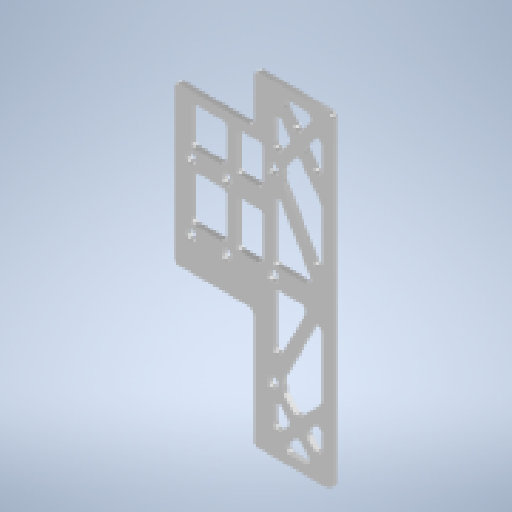
# Autodesk Inventor part: base2fork_connecter_front
Saved by Autodesk Inventor 2024.1 (Build 281209000, 209)
## iProperties
Created: 2025-03-04
Part Number: base2fork_connecter_front
Material: アルミニウム 6061
Document SubType Name: Sheet Metal
Designer: hibik
Density: 2.7 g/cm^3
Sheet Metal Rule: Default_mm
Appearance: アルミニウム - フラット
Author: hibik
Autodesk Inventor part; units mm, degrees
ref_plane "YZ Plane" through (0, 0, 0) normal (1, 0, 0) x (0, 1, 0)
ref_plane "XZ Plane" through (0, 0, 0) normal (0, 1, 0) x (-1, 0, 0)
ref_plane "XY Plane" through (0, 0, 0) normal (0, 0, 1) x (1, 0, 0)
sketch "スケッチ1 outline for プレート1" plane through (0, 0, 0) normal (0, 0, 1) x (1, 0, 0)
  line L0 (11.969655, 0) -> (24.990381, 0)
  line L1 (4.255354, 0) -> (11.969655, 0)
  line L2 (24.990381, 0) -> (24.990381, 47.7)
  line L3 (4.255354, 47.7) -> (4.255354, 0)
  line L4 (24.990381, 47.7) -> (13.490381, 47.7)
  line L5 (13.490381, 47.7) -> (4.255354, 47.7)
  circle A0 centre (9.255354, 10) radius 1.6
  circle A1 centre (19.990381, 10) radius 1.6
  circle A2 centre (9.255354, 30) radius 1.6
  circle A3 centre (19.990381, 30) radius 1.6
extrude "プレート1" add sketch "スケッチ1 outline for プレート1" along normal blind 1.5
sketch "スケッチ2 outline for プレート2" plane through (0, 0, 1.5) normal (0, 0, 1) x (1, 0, 0)
  line L0 (28.216878, 0) -> (28.216878, -35.8)
  line L1 (28.216878, -35.8) -> (51.990381, -35.8)
  line L2 (51.990381, -35.8) -> (51.990381, 62.7)
  line L3 (51.990381, 62.7) -> (28.216878, 62.7)
  line L4 (28.216878, 62.7) -> (28.216878, 47.7)
  line L5 (28.216878, 47.7) -> (24.990381, 47.7)
  line L6 (24.990381, 47.7) -> (24.990381, 0)
  line L7 (24.990381, 0) -> (28.216878, 0)
  circle A0 centre (33.990381, -16.45) radius 1.6
  circle A1 centre (33.990381, 39.55) radius 1.6
  circle A2 centre (33.990381, 11.55) radius 1.6
sheet face with bend "面2" sketch "スケッチ2 outline for プレート2" thickness 1.5 toward (0, 0, -1) bend radius 1.5
bend "曲げ1"
sketch "スケッチ1" plane through (0, 0, 0) normal (0, 0, 1) x (1, 0, 0)
  circle A0 centre (9.255354, 10) radius 1.6
  circle A1 centre (19.990381, 30) radius 1.6
  circle A2 centre (9.255354, 30) radius 1.6
  circle A3 centre (19.990381, 50) radius 1.6
  circle A4 centre (19.990381, 10) radius 1.6
  line L0 (13.490381, 47.7) -> (-5.744646, 47.7)
  line L1 (-5.744646, 47.7) -> (-5.744646, 0)
  line L2 (0, 0) -> (-5.744646, 0)
  line L3 (0, -16) -> (0, 0)
  line L4 (0, -16) -> (11.969655, -16)
  line L5 (11.969655, 0) -> (11.969655, -16)
  line L6 (24.990381, 0) -> (11.969655, 0)
  line L7 (24.990381, 62.7) -> (24.990381, 0)
  line L8 (13.490381, 62.7) -> (24.990381, 62.7)
  line L9 (13.490381, 62.7) -> (13.490381, 47.7)
  line L10 (0, 0) -> (11.969655, 0)
  line L11 (4.255354, 47.7) -> (4.255354, 0)
  line L12 (13.490381, 47.7) -> (24.990381, 47.7)
  dimension "d0" = 5
  dimension "d1" = 15
  dimension "d2" = 20
  dimension "d3" = 20
  dimension "d4" = 10
  dimension "d5" = 30.73503
  dimension "d6" = 78.7
  dimension "d7" = 62.7
  dimension "d8" = 19.23503
  dimension "d9" = 11.96966
  dimension "d10" = 5.74465
  dimension "d11" = 15
  dimension "d12" = 3.2
  dimension "d14" = 5
  measures "d0" distance from line of L7 A3.centre
  measures "d1" distance from line of L1 A2.centre
  measures "d2" distance of A1.centre A3.centre
  measures "d3" distance of A4.centre A1.centre
  measures "d4" distance from line of L6 A4.centre
  measures "d5" distance between parallel lines of L1 L7
  measures "d6" distance between parallel lines of L4 L8
  measures "d7" distance of L7.start L6.start
  measures "d8" distance of L0.start L0.end
  measures "d9" distance of L3.start L4.end
  measures "d10" distance of L2.start L1.end
  measures "d11" distance of L8.start L0.start
  measures "d12" diameter of A3
  measures "d14" distance from line of L11 A2.centre
sketch "スケッチ2" plane through (0, 0, 1.5) normal (0, 0, 1) x (1, 0, 0)
  circle A0 centre (33.990381, 39.55) radius 1.6
  circle A1 centre (33.990381, 11.55) radius 1.6
  circle A2 centre (33.990381, -16.45) radius 1.6
  line L0 (28.216878, -34.3) -> (51.990381, -34.3)
  line L1 (51.990381, -34.3) -> (51.990381, 62.7)
  line L2 (28.216878, 62.7) -> (51.990381, 62.7)
  line L3 (28.216878, -34.3) -> (28.216878, 62.7)
  line L4 (39.417474, -31.3) -> (32.835681, -31.3)
  line L5 (32.835681, -31.3) -> (32.835681, -27.3)
  line L6 (32.835681, -27.3) -> (39.417474, -27.3)
  line L7 (39.417474, -27.3) -> (39.417474, -31.3)
  line L8 (39.417474, 59.7) -> (39.417474, 55.7)
  line L9 (39.417474, 55.7) -> (32.835681, 55.7)
  line L10 (32.835681, 55.7) -> (32.835681, 59.7)
  line L11 (39.417474, 59.7) -> (32.835681, 59.7)
  line L12 (24.990381, 47.7) -> (24.990381, 0)
  line L13 (24.990381, 0) -> (28.216878, 0)
  line L14 (28.216878, -34.3) -> (51.990381, -34.3)
  line L15 (51.990381, -34.3) -> (51.990381, -35.8)
  line L16 (51.990381, -35.8) -> (28.216878, -35.8)
  line L17 (28.216878, -35.8) -> (28.216878, -34.3)
  line L18 (30.216878, 0) -> (30.216878, -35.8)
  line L19 (4.255354, 0) -> (24.990381, 0)
  line L20 (24.990381, 0) -> (30.216878, 0)
  line L21 (24.990381, 47.7) -> (28.216878, 47.7)
  point P0 (0, 0)
  point P1 (30.216878, -34.3)
  dimension "d21" = 1.5
  dimension "d25" = 2
  measures "d21" distance of L14.end L15.end
  measures "d25" distance between parallel lines of L3 L18
fillet "フィレット1" radius 1.5 4 edges at (4.2554, 0, 0.75) (4.2554, 47.7, 0.75) (51.9904, 62.7, 0.75) (51.9904, -35.8, 0.75)
sketch "スケッチ3" plane through (0, 0, 1.5) normal (0, 0, 1) x (1, 0, 0)
  arc A0 (5.755354, 47.7) -> (4.255354, 46.2) centre (5.755354, 46.2) ccw
  line L0 (4.255354, 1.5) -> (4.255354, 46.2)
  arc A1 (4.255354, 1.5) -> (5.755354, 0) centre (5.755354, 1.5) ccw
  line L1 (28.216878, 0) -> (5.755354, 0)
  circle A2 centre (19.990381, 10) radius 1.6
  circle A3 centre (9.255354, 30) radius 1.6
  circle A4 centre (19.990381, 30) radius 1.6
  circle A5 centre (9.255354, 10) radius 1.6
  line L2 (19.990381, 10) -> (9.255354, 10)
  line L3 (9.255354, 10) -> (9.255354, 44.7)
  line L4 (9.255354, 44.7) -> (19.990381, 44.7)
  line L5 (19.990381, 44.7) -> (19.990381, 10)
  circle A6 centre (9.255354, 30) radius 3
  circle A7 centre (19.990381, 30) radius 3
  circle A8 centre (19.990381, 10) radius 3
  circle A9 centre (9.255354, 10) radius 3
  line L6 (33.990381, 59.7) -> (48.990381, 59.7)
  line L7 (48.990381, 59.7) -> (48.990381, -32.8)
  line L8 (48.990381, -32.8) -> (33.990381, -32.8)
  line L9 (33.990381, -32.8) -> (33.990381, 59.7)
  line L10 (32.885071, -31.785954) -> (35.095691, -33.814046)
  line L11 (35.095691, -33.814046) -> (50.095691, -17.464046)
  line L12 (50.095691, -17.464046) -> (47.885071, -15.435954)
  line L13 (47.885071, -15.435954) -> (32.885071, -31.785954)
  line L14 (47.885071, -33.814046) -> (50.095691, -31.785954)
  line L15 (50.095691, -31.785954) -> (35.095691, -15.435954)
  line L16 (35.095691, -15.435954) -> (32.885071, -17.464046)
  line L17 (32.885071, -17.464046) -> (47.885071, -33.814046)
  line L18 (32.649638, -15.777387) -> (35.331124, -17.122613)
  line L19 (35.331124, -17.122613) -> (50.331124, 12.777387)
  line L20 (50.331124, 12.777387) -> (47.649638, 14.122613)
  line L21 (47.649638, 14.122613) -> (32.649638, -15.777387)
  line L22 (47.68986, 12.702574) -> (50.290902, 14.197426)
  line L23 (50.290902, 14.197426) -> (35.290902, 40.297426)
  line L24 (35.290902, 40.297426) -> (32.68986, 38.802574)
  line L25 (32.68986, 38.802574) -> (47.68986, 12.702574)
  line L26 (32.787164, 40.445695) -> (35.193598, 38.654305)
  line L27 (35.193598, 38.654305) -> (50.193598, 58.804305)
  line L28 (50.193598, 58.804305) -> (47.787164, 60.595695)
  line L29 (47.787164, 60.595695) -> (32.787164, 40.445695)
  circle A10 centre (33.990381, 11.55) radius 3
  circle A11 centre (33.990381, 39.55) radius 3
  circle A12 centre (33.990381, -16.45) radius 3
  line L30 (35.193598, 60.595695) -> (32.787164, 58.804305)
  line L31 (32.787164, 58.804305) -> (47.787164, 38.654305)
  line L32 (47.787164, 38.654305) -> (50.193598, 40.445695)
  line L33 (50.193598, 40.445695) -> (35.193598, 60.595695)
  line L34 (47.787164, 38.654305) -> (48.990381, 37.037984)
  line L35 (47.885071, -15.435954) -> (48.990381, -14.231166)
  line L36 (33.990381, 14.55) -> (48.990381, 14.55)
  line L37 (48.990381, 14.55) -> (48.990381, 8.55)
  line L38 (48.990381, 8.55) -> (33.990381, 8.55)
  line L39 (33.990381, 8.55) -> (33.990381, 14.55)
  line L40 (5.755354, 0) -> (28.216878, 0)
  line L41 (9.255354, 33) -> (19.990381, 33)
  line L42 (19.990381, 33) -> (19.990381, 27)
  line L43 (19.990381, 27) -> (9.255354, 27)
  line L44 (9.255354, 27) -> (9.255354, 33)
  line L45 (9.255354, 13) -> (19.990381, 13)
  line L46 (22.990381, 0) -> (22.990381, 40.319398)
  line L47 (22.990381, 3) -> (28.716878, 3)
  line L48 (19.990381, 33) -> (30.990381, 33)
  line L49 (30.990381, 33) -> (30.990381, 27)
  line L50 (30.990381, 27) -> (19.990381, 27)
  line L51 (19.990381, 27) -> (19.990381, 33)
  line L52 (19.990381, 13) -> (30.990381, 13)
  line L53 (30.990381, 13) -> (30.990381, 7)
  line L54 (30.990381, 7) -> (19.990381, 7)
  line L55 (19.990381, 7) -> (19.990381, 13)
  line L56 (22.990381, 40.319398) -> (22.990381, 49.080602)
  line L57 (28.216878, -35.8) -> (50.490381, -35.8)
  arc A13 (50.490381, -35.8) -> (51.990381, -34.3) centre (50.490381, -34.3) ccw
  line L58 (51.990381, -34.3) -> (51.990381, 61.2)
  arc A14 (51.990381, 61.2) -> (50.490381, 62.7) centre (50.490381, 61.2) ccw
  line L59 (50.490381, 62.7) -> (28.216878, 62.7)
  line L60 (28.216878, 62.7) -> (28.216878, 47.7)
  line L61 (28.216878, 47.7) -> (5.755354, 47.7)
  line L62 (28.216878, 0) -> (28.216878, -35.8)
  line L63 (30.990381, 39.55) -> (30.990381, 11.55)
  circle A15 centre (33.990381, 39.55) radius 1.6
  circle A16 centre (33.990381, 11.55) radius 1.6
  circle A17 centre (33.990381, -16.45) radius 1.6
  line L64 (30.990381, 13) -> (31.364072, 13)
  line L65 (19.990381, 44.7) -> (30.990381, 44.7)
  line L66 (30.990381, 44.7) -> (30.990381, 39.55)
  line L67 (30.990381, 44.7) -> (30.990381, 59.7)
  line L68 (30.990381, 59.7) -> (33.990381, 59.7)
  point P0 (0, 0)
  point P1 (28.716878, 0)
  point P2 (48.990381, 13.45)
  point P3 (48.990381, -16.45)
  point P4 (77.261765, 39.55)
  point P5 (43.526009, -24.625)
  point P6 (48.990381, -30.581166)
  point P7 (48.990381, -18.668834)
  point P8 (46.954753, -32.8)
  point P9 (41.490381, -26.843834)
  point P10 (36.026009, -32.8)
  point P11 (34.64145, -19.378499)
  point P12 (33.990381, -19.45)
  point P13 (33.990381, -30.581166)
  point P14 (39.454753, -24.625)
  point P15 (48.210361, 8.55)
  point P16 (36.496124, -14.800379)
  point P17 (36.852071, -17.350407)
  point P18 (41.490381, -22.406166)
  point P19 (44.854013, 8.55)
  point P20 (33.990381, 8.55)
  point P21 (33.990381, -13.104839)
  point P22 (46.628121, 14.55)
  point P23 (33.990381, 36.539668)
  point P24 (41.490381, 47.112984)
  point P25 (36.744987, 40.738338)
  point P26 (36.585481, 38.044858)
  point P27 (48.990381, 16.460332)
  point P28 (39.620394, 49.625)
  point P29 (33.990381, 57.187984)
  point P30 (33.990381, 42.55)
  point P31 (34.338553, 42.529728)
  point P32 (43.360368, 49.625)
  point P33 (48.990381, 42.062016)
  point P34 (48.990381, 57.187984)
  point P35 (35.860368, 59.7)
  point P36 (41.490381, 52.137016)
  point P37 (47.120394, 59.7)
  point P38 (9.255354, 27)
  point P39 (19.990381, 33)
  point P40 (22.990381, 33)
  point P41 (22.990381, 7)
  point P42 (22.990381, 13)
  point P43 (22.990381, 27)
  point P44 (24.990381, 0)
  point P45 (33.990381, 42.062016)
  point P46 (22.990381, 44.7)
  point P47 (19.990381, 31.6)
  point P48 (19.990381, 28.4)
  point P49 (33.990381, 9.95)
  point P50 (33.990381, 13.15)
  point P51 (32.899302, -15.279724)
  point P52 (33.990381, -16.45)
  point P53 (33.990381, -18.05)
  point P54 (35.580787, -16.624951)
  point P55 (35.79492, -16.198113)
  point P56 (35.472089, -15.846228)
  point P57 (19.990381, 8.4)
  point P58 (19.990381, 11.6)
  point P59 (35.526066, 39.10092)
  point P60 (35.781413, 39.443937)
  point P61 (35.568335, 39.814693)
  point P62 (33.990381, 41.15)
  point P63 (32.967293, 38.319841)
  point P64 (33.990381, 36.55)
  point P65 (33.98444, 36.550006)
  point P66 (33.814639, -13.455152)
  point P67 (33.990381, -13.45)
  dimension "d27" = 6
  dimension "d32" = 6
  dimension "d33" = 6
  dimension "d34" = 6
  dimension "d35" = 3
  dimension "d39" = 3
  dimension "d42" = 3
  dimension "d43" = 3
  dimension "d44" = 3
  dimension "d45" = 3
  constraints: 120 end point, 25 parallel, 15 perpendicular, 15 point on line, 12 midpoint, 9 horizontal, 8 tangent, 6 coincident, 5 centre point, 5 equal length, 5 point on circle, 3 concentric, 2 horizontal alignment, 2 vertical, 2 vertical alignment, 1 collinear, 1 equal radius, 5 other
  measures "d27" diameter of A6
  measures "d32" diameter of A10
  measures "d33" diameter of A11
  measures "d34" diameter of A12
  measures "d35" distance between parallel lines of L27 L29
  measures "d39" distance between parallel lines of L1 L47
  measures "d42" distance between parallel lines of L61 L4
  measures "d43" distance between parallel lines of L58 L7
  measures "d44" distance between parallel lines of L59 L6
  measures "d45" distance between parallel lines of L57 L8
sketch "スケッチ3 outline for 押し出し1" plane through (0, 0, 1.5) normal (0, 0, 1) x (1, 0, 0)
  line L0 (43.360368, 49.625) -> (48.990381, 42.062016)
  line L1 (48.990381, 57.187984) -> (43.360368, 49.625)
  line L2 (48.990381, 42.062016) -> (48.990381, 57.187984)
  line L3 (9.255354, 13) -> (19.990381, 13)
  line L4 (9.255354, 27) -> (9.255354, 13)
  line L5 (19.990381, 27) -> (9.255354, 27)
  line L6 (19.990381, 13) -> (19.990381, 27)
  line L7 (19.990381, 44.7) -> (9.255354, 44.7)
  line L8 (19.990381, 33) -> (19.990381, 44.7)
  line L9 (9.255354, 33) -> (19.990381, 33)
  line L10 (9.255354, 44.7) -> (9.255354, 33)
  line L11 (30.990381, 13) -> (30.990381, 27)
  line L12 (22.990381, 13) -> (30.990381, 13)
  line L13 (22.990381, 27) -> (22.990381, 13)
  line L14 (30.990381, 27) -> (22.990381, 27)
  line L15 (30.990381, 33) -> (30.990381, 44.7)
  line L16 (30.990381, 44.7) -> (22.990381, 44.7)
  line L17 (22.990381, 44.7) -> (22.990381, 33)
  line L18 (22.990381, 33) -> (30.990381, 33)
  line L19 (19.990381, 31.6) -> (19.990381, 28.4)
  arc A0 (19.990381, 28.4) -> (19.990381, 31.6) centre (19.990381, 30) ccw
  line L20 (39.620394, 49.625) -> (33.990381, 57.187984)
  line L21 (34.338553, 42.529728) -> (39.620394, 49.625)
  arc A1 (33.990381, 42.55) -> (34.338553, 42.529728) centre (33.990381, 39.55) cw
  line L22 (33.990381, 57.187984) -> (33.990381, 42.55)
  arc A2 (33.990381, 9.95) -> (33.990381, 13.15) centre (33.990381, 11.55) ccw
  line L23 (33.990381, 13.15) -> (33.990381, 9.95)
  line L24 (19.990381, 11.6) -> (19.990381, 8.4)
  arc A3 (19.990381, 8.4) -> (19.990381, 11.6) centre (19.990381, 10) ccw
  line L25 (35.860368, 59.7) -> (41.490381, 52.137016)
  line L26 (47.120394, 59.7) -> (35.860368, 59.7)
  line L27 (41.490381, 52.137016) -> (47.120394, 59.7)
  line L28 (48.990381, 37.037984) -> (41.490381, 47.112984)
  line L29 (41.490381, 47.112984) -> (36.744987, 40.738338)
  arc A4 (36.744987, 40.738338) -> (36.585481, 38.044858) centre (33.990381, 39.55) cw
  line L30 (36.585481, 38.044858) -> (48.990381, 16.460332)
  line L31 (48.990381, 16.460332) -> (48.990381, 37.037984)
  line L32 (33.990381, 14.55) -> (46.628121, 14.55)
  line L33 (33.990381, 36.539668) -> (33.990381, 14.55)
  line L34 (46.628121, 14.55) -> (33.990381, 36.539668)
  line L35 (44.854013, 8.55) -> (33.990381, 8.55)
  line L36 (33.990381, -13.104839) -> (44.854013, 8.55)
  line L37 (33.990381, 8.55) -> (33.990381, -13.104839)
  line L38 (48.990381, 8.55) -> (48.210361, 8.55)
  line L39 (48.210361, 8.55) -> (36.496124, -14.800379)
  arc A5 (36.496124, -14.800379) -> (36.852071, -17.350407) centre (33.990381, -16.45) cw
  line L40 (36.852071, -17.350407) -> (41.490381, -22.406166)
  line L41 (41.490381, -22.406166) -> (48.990381, -14.231166)
  line L42 (48.990381, -14.231166) -> (48.990381, 8.55)
  arc A6 (34.64145, -19.378499) -> (33.990381, -19.45) centre (33.990381, -16.45) cw
  line L43 (39.454753, -24.625) -> (34.64145, -19.378499)
  line L44 (33.990381, -30.581166) -> (39.454753, -24.625)
  line L45 (33.990381, -19.45) -> (33.990381, -30.581166)
  line L46 (46.954753, -32.8) -> (41.490381, -26.843834)
  line L47 (36.026009, -32.8) -> (46.954753, -32.8)
  line L48 (41.490381, -26.843834) -> (36.026009, -32.8)
  line L49 (43.526009, -24.625) -> (48.990381, -30.581166)
  line L50 (48.990381, -18.668834) -> (43.526009, -24.625)
  line L51 (48.990381, -30.581166) -> (48.990381, -18.668834)
  arc A7 (33.990381, -18.05) -> (32.899302, -15.279724) centre (33.990381, -16.45) ccw
  line L52 (33.990381, -16.45) -> (33.990381, -18.05)
  line L53 (32.649638, -15.777387) -> (33.990381, -16.45)
  line L54 (32.899302, -15.279724) -> (32.649638, -15.777387)
  arc A8 (32.967293, 38.319841) -> (33.990381, 41.15) centre (33.990381, 39.55) ccw
  line L55 (32.68986, 38.802574) -> (32.967293, 38.319841)
  line L56 (33.990381, 39.55) -> (32.68986, 38.802574)
  line L57 (33.990381, 41.15) -> (33.990381, 39.55)
extrude "押し出し1" cut sketch "スケッチ3 outline for 押し出し1" against normal through all
fillet "フィレット2" radius 1.5 41 edges at (9.2554, 13, 0.75) (22.9904, 13, 0.75) (33.9904, 14.55, 0.75) (22.9904, 33, 0.75) (9.2554, 33, 0.75) (41.4904, 52.137, 0.75) (33.9904, -13.1048, 0.75) (33.9904, -30.5812, 0.75) (36.026, -32.8, 0.75) (41.4904, -22.4062, 0.75) (36.8521, -17.3504, 0.75) (36.4961, -14.8004, 0.75) (48.9904, -30.5812, 0.75) (43.526, -24.625, 0.75) (48.9904, -18.6688, 0.75) (41.4904, -26.8438, 0.75) (46.9548, -32.8, 0.75) (39.4548, -24.625, 0.75) (34.6415, -19.3785, 0.75) (33.9904, -19.45, 0.75) (48.9904, -14.2312, 0.75) (48.9904, 8.55, 0.75) (48.2104, 8.55, 0.75) (44.854, 8.55, 0.75) (33.9904, 8.55, 0.75) (46.6281, 14.55, 0.75) (48.9904, 16.4603, 0.75) (48.9904, 37.038, 0.75) (48.9904, 42.062, 0.75) (43.3604, 49.625, 0.75) (48.9904, 57.188, 0.75) (47.1204, 59.7, 0.75) (35.8604, 59.7, 0.75) (33.9904, 57.188, 0.75) (19.9904, 44.7, 0.75) (19.9904, 33, 0.75) (9.2554, 44.7, 0.75) (9.2554, 27, 0.75) (19.9904, 27, 0.75) (22.9904, 27, 0.75) (19.9904, 13, 0.75)
fillet "フィレット4" radius 1.5 16 edges at (39.6204, 49.625, 0.75) (41.4904, 47.113, 0.75) (36.5855, 38.0449, 0.75) (36.745, 40.7383, 0.75) (33.9904, 36.5397, 0.75) (30.9904, 44.7, 0.75) (30.9904, 33, 0.75) (30.9904, 27, 0.75) (30.9904, 13, 0.75) (22.9904, 44.7, 0.75) (33.9904, 42.55, 0.75) (34.3386, 42.5297, 0.75) (28.2169, 0, 0.75) (28.2169, -35.8, 0.75) (28.2169, 47.7, 0.75) (28.2169, 62.7, 0.75)
equation "\"d14\" = d0"
equation "\"d39\" = d26"
equation "\"d13\" = Thickness"
equation "\"d15\" = BendRadius"
equation "\"d16\" = BendReliefWidth"
equation "\"d18\" = MinimumRemnant"
equation "\"d17\" = BendReliefDepth"
equation "\"d19\" = TransitionRadius"
equation "\"BendRadius\" = Thickness"
equation "\"BendReliefWidth\" = Thickness"
equation "\"BendReliefDepth\" = 0.5 * Thickness"
equation "\"CornerReliefSize\" = 4 * Thickness"
equation "\"MinimumRemnant\" = 2 * Thickness"
equation "\"TransitionRadius\" = BendRadius"
equation "\"JacobiRadiusSize\" = BendRadius"
equation "\"GapSize\" = Thickness"
equation "\"d26\" = 3"
equation "\"Thickness\" = 1.5"
